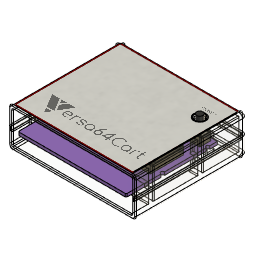
versa64case_2_0_closed v9 (Autodesk Fusion 360 design; units mm, degrees)
Autodesk Fusion 360 part; units mm, degrees
(part 1 of 2)
sketch "Versa64Cart_v1_6" plane through (0, 0, 0) normal (0, 0, 1) x (1, 0, 0) in component "Versa64cart_v1.6"
  line L0 (0, 11) -> (0, 18.6)
  line L1 (0, 20.6) -> (0, 42.9)
  line L2 (0, 44.9) -> (0, 48.9)
  line L3 (0, 48.9) -> (58, 48.9)
  line L4 (58, 48.9) -> (58, 44.8)
  line L5 (58, 42.9) -> (58, 20.6)
  line L6 (58, 18.6) -> (58, 11)
  arc A0 (0, 18.6) -> (1, 19.6) centre (0, 19.6) ccw
  arc A1 (1, 19.6) -> (0, 20.6) centre (0, 19.6) ccw
  arc A2 (0, 42.9) -> (1, 43.9) centre (0, 43.9) ccw
  arc A3 (1, 43.9) -> (0, 44.9) centre (0, 43.9) ccw
  arc A4 (57, 19.6) -> (58, 18.6) centre (58, 19.6) ccw
  arc A5 (58, 20.6) -> (57, 19.6) centre (58, 19.6) ccw
  line L7 (58, 42.9) -> (57.9, 42.9)
  arc A6 (57, 43.8) -> (57.9, 42.9) centre (57.9, 43.8) ccw
  arc A7 (58, 44.8) -> (57, 43.8) centre (58, 43.8) ccw
  circle A8 centre (29, 43.9) radius 2.5
  line L8 (57.5, 0) -> (0.5, 0)
  line L9 (0.5, 0) -> (0, 0.5)
  line L10 (0, 0.5) -> (0, 11)
  line L11 (57.5, 0) -> (58, 0.5)
  line L12 (58, 0.5) -> (58, 11)
  line L13 (19.4945, 23.3362) -> (19.4945, 18.0023) construction
  arc A9 (19.4945, 23.3363) -> (19.4945, 25.8763) centre (19.4945, 24.6063) ccw construction
  line L14 (54.8005, 18.0023) -> (54.8005, 31.2103) construction
  line L15 (19.4945, 31.2103) -> (19.4945, 25.8763) construction
  line L16 (19.4945, 31.2103) -> (54.8005, 31.2103) construction
  line L17 (19.4945, 18.0023) -> (54.8005, 18.0023) construction
  line L18 (41.7512, 46.99) -> (43.0213, 46.99)
  line L19 (43.0213, 46.99) -> (43.3388, 46.6725)
  line L20 (43.3388, 44.7675) -> (43.0213, 44.45)
  line L21 (41.1163, 46.355) -> (41.1163, 45.085)
  line L22 (41.7512, 46.99) -> (41.1163, 46.355)
  line L23 (41.1163, 45.085) -> (41.1163, 44.45)
  line L24 (43.0213, 44.45) -> (41.1163, 44.45)
  line L25 (43.9738, 46.6725) -> (44.2913, 46.99)
  line L26 (44.2913, 46.99) -> (45.5613, 46.99)
  line L27 (45.5613, 44.45) -> (44.2913, 44.45)
  line L28 (44.2913, 44.45) -> (43.9738, 44.7675)
  line L29 (44.2913, 46.99) -> (45.5613, 46.99)
  line L30 (45.5613, 46.99) -> (45.8788, 46.6725)
  line L31 (45.8788, 44.7675) -> (45.5613, 44.45)
  line L32 (46.5138, 46.6725) -> (46.8313, 46.99)
  line L33 (46.8313, 46.99) -> (48.1013, 46.99)
  line L34 (48.1013, 46.99) -> (48.7363, 46.355)
  line L35 (48.7363, 46.355) -> (48.7363, 45.085)
  line L36 (48.7363, 45.085) -> (48.1013, 44.45)
  line L37 (48.1013, 44.45) -> (46.8313, 44.45)
  line L38 (46.8313, 44.45) -> (46.5138, 44.7675)
  line L39 (40.64, 45.8788) -> (40.7988, 46.0375)
  line L40 (40.7988, 46.0375) -> (40.7988, 45.4025)
  line L41 (40.64, 45.4025) -> (40.9575, 45.4025)
  line L42 (40.64, 46.99) -> (40.64, 44.45)
  line L43 (40.005, 46.99) -> (38.735, 46.99)
  line L44 (40.64, 46.99) -> (40.005, 46.99)
  line L45 (38.735, 46.99) -> (38.1, 46.355)
  line L46 (38.1, 44.45) -> (38.1, 46.355)
  line L47 (40.64, 44.45) -> (40.64, 42.545)
  line L48 (40.64, 42.545) -> (40.005, 41.91)
  line L49 (40.005, 41.91) -> (38.735, 41.91)
  line L50 (38.735, 41.91) -> (38.1, 42.545)
  line L51 (38.1, 42.545) -> (38.1, 44.45)
  line L52 (38.1, 46.355) -> (38.1, 44.45)
  line L53 (37.465, 46.99) -> (36.195, 46.99)
  line L54 (38.1, 46.355) -> (37.465, 46.99)
  line L55 (36.195, 46.99) -> (35.56, 46.355)
  line L56 (35.56, 43.815) -> (35.56, 46.355)
  line L57 (38.1, 44.45) -> (38.1, 42.545)
  line L58 (38.1, 42.545) -> (37.465, 41.91)
  line L59 (37.465, 41.91) -> (36.195, 41.91)
  line L60 (36.195, 41.91) -> (35.56, 42.545)
  line L61 (35.56, 42.545) -> (35.56, 43.815)
  line L62 (34.925, 46.99) -> (33.655, 46.99)
  line L63 (35.56, 46.355) -> (34.925, 46.99)
  line L64 (33.655, 46.99) -> (33.02, 46.355)
  line L65 (33.02, 43.815) -> (33.02, 46.355)
  line L66 (35.56, 42.545) -> (34.925, 41.91)
  line L67 (34.925, 41.91) -> (33.655, 41.91)
  line L68 (33.655, 41.91) -> (33.02, 42.545)
  line L69 (33.02, 42.545) -> (33.02, 43.815)
  line L70 (1.6193, 35.8458) -> (15.8433, 35.8458)
  line L71 (15.8433, 45.7518) -> (1.6193, 45.7518)
  line L72 (1.6193, 45.7518) -> (1.6193, 42.4498)
  line L73 (1.6193, 39.1478) -> (2.1273, 39.1478)
  line L74 (2.1273, 39.1478) -> (2.1273, 42.4498)
  line L75 (2.1273, 42.4498) -> (1.6193, 42.4498)
  line L76 (1.6193, 39.1478) -> (1.6193, 35.8458)
  line L77 (1.6193, 42.4498) -> (1.6193, 39.1478)
  line L78 (15.8433, 35.8458) -> (15.8433, 39.1478)
  line L79 (15.8433, 42.4498) -> (15.3353, 42.4498)
  line L80 (15.3353, 42.4498) -> (15.3353, 39.1478)
  line L81 (15.3353, 39.1478) -> (15.8433, 39.1478)
  line L82 (15.8433, 42.4498) -> (15.8433, 45.7518)
  line L83 (15.8433, 39.1478) -> (15.8433, 42.4498)
  line L84 (2.8893, 41.6878) -> (2.8893, 38.8938)
  line L85 (4.4133, 38.8938) -> (4.4133, 41.6878)
  line L86 (4.4133, 38.8938) -> (2.8893, 38.8938)
  line L87 (3.1433, 40.7988) -> (3.1433, 39.1478)
  line L88 (4.1593, 40.7988) -> (4.1593, 39.1478)
  line L89 (2.8893, 42.4498) -> (2.8893, 42.7037)
  line L90 (2.8893, 42.7037) -> (3.1433, 42.7037)
  line L91 (4.1593, 42.7037) -> (4.4133, 42.7037)
  line L92 (4.4133, 42.7037) -> (4.4133, 42.4498)
  line L93 (5.4293, 41.6878) -> (5.4293, 38.8938)
  line L94 (6.9533, 38.8938) -> (6.9533, 41.6878)
  line L95 (6.9533, 38.8938) -> (5.4293, 38.8938)
  line L96 (5.6833, 40.7988) -> (5.6833, 39.1478)
  line L97 (6.6993, 40.7988) -> (6.6993, 39.1478)
  line L98 (5.4293, 42.4498) -> (5.4293, 42.7037)
  line L99 (5.4293, 42.7037) -> (5.6833, 42.7037)
  line L100 (6.6993, 42.7037) -> (6.9533, 42.7037)
  line L101 (6.9533, 42.7037) -> (6.9533, 42.4498)
  line L102 (7.9693, 41.6878) -> (7.9693, 38.8938)
  line L103 (9.4932, 38.8938) -> (9.4932, 41.6878)
  line L104 (9.4932, 38.8938) -> (7.9693, 38.8938)
  line L105 (8.2233, 40.7988) -> (8.2233, 39.1478)
  line L106 (9.2393, 40.7988) -> (9.2393, 39.1478)
  line L107 (7.9693, 42.4498) -> (7.9693, 42.7037)
  line L108 (7.9693, 42.7037) -> (8.2233, 42.7037)
  line L109 (9.2393, 42.7037) -> (9.4932, 42.7037)
  line L110 (9.4932, 42.7037) -> (9.4932, 42.4498)
  line L111 (10.5092, 41.6878) -> (10.5092, 38.8938)
  line L112 (12.0333, 38.8938) -> (12.0333, 41.6878)
  line L113 (12.0333, 38.8938) -> (10.5092, 38.8938)
  line L114 (10.7633, 40.7988) -> (10.7633, 39.1478)
  line L115 (11.7793, 40.7988) -> (11.7793, 39.1478)
  line L116 (10.5092, 42.4498) -> (10.5092, 42.7037)
  line L117 (10.5092, 42.7037) -> (10.7633, 42.7037)
  line L118 (11.7793, 42.7037) -> (12.0333, 42.7037)
  line L119 (12.0333, 42.7037) -> (12.0333, 42.4498)
  line L120 (13.0493, 41.6878) -> (13.0493, 38.8938)
  line L121 (14.5732, 38.8938) -> (14.5732, 41.6878)
  line L122 (14.5732, 38.8938) -> (13.0493, 38.8938)
  line L123 (13.3033, 40.7988) -> (13.3033, 39.1478)
  line L124 (14.3193, 40.7988) -> (14.3193, 39.1478)
  line L125 (13.0493, 42.4498) -> (13.0493, 42.7037)
  line L126 (13.0493, 42.7037) -> (13.3033, 42.7037)
  line L127 (14.3193, 42.7037) -> (14.5732, 42.7037)
  line L128 (14.5732, 42.7037) -> (14.5732, 42.4498)
  line L129 (55.65, 41.6) -> (50.15, 41.6)
  line L130 (49.9, 43.15) -> (49.9, 46)
  line L131 (50.5, 47.6) -> (55.65, 47.6)
  line L132 (55.9, 46.05) -> (55.9, 43.15)
  arc A10 (55.35, 47.15) -> (55.4, 46.4) centre (55.0498, 46.7533) ccw
  arc A11 (55.35, 42.85) -> (55.4, 42.1) centre (55.0498, 42.4533) ccw
  arc A12 (50.45, 42.05) -> (50.4, 42.8) centre (50.7502, 42.4467) ccw
  arc A13 (50.45, 46.35) -> (50.45, 47.15) centre (50.75, 46.75) ccw
  circle A14 centre (52.9, 44.6) radius 1.75
  circle A15 centre (52.9, 44.6) radius 1.4
  line L133 (9.2393, 39.7828) -> (9.2393, 40.1638)
  line L134 (5.6833, 39.7828) -> (6.6993, 39.7828)
  line L135 (4.1593, 40.1638) -> (3.1433, 40.1638)
  line L136 (5.6833, 40.4178) -> (6.6993, 40.4178)
  line L137 (11.7793, 39.1478) -> (11.7793, 39.5288)
  line L138 (6.6993, 40.1638) -> (5.6833, 40.1638)
  line L139 (3.1433, 39.5288) -> (3.1433, 39.1478)
  line L140 (4.1593, 40.7988) -> (3.1433, 40.7988)
  line L141 (8.2233, 39.7828) -> (9.2393, 39.7828)
  line L142 (11.7793, 39.7828) -> (11.7793, 40.1638)
  line L143 (10.7633, 40.4178) -> (11.7793, 40.4178)
  line L144 (3.1433, 40.7988) -> (3.1433, 40.4178)
  line L145 (6.6993, 40.4178) -> (6.6993, 40.7988)
  line L146 (6.6993, 39.5288) -> (5.6833, 39.5288)
  line L147 (9.2393, 40.1638) -> (8.2233, 40.1638)
  line L148 (6.6993, 40.7988) -> (5.6833, 40.7988)
  line L149 (11.7793, 40.1638) -> (10.7633, 40.1638)
  line L150 (11.7793, 40.7988) -> (10.7633, 40.7988)
  line L151 (9.2393, 40.4178) -> (9.2393, 40.7988)
  line L152 (9.2393, 39.5288) -> (8.2233, 39.5288)
  line L153 (3.1433, 39.1478) -> (4.1593, 39.1478)
  line L154 (4.1593, 40.4178) -> (4.1593, 40.7988)
  line L155 (10.7633, 39.7828) -> (11.7793, 39.7828)
  line L156 (3.1433, 40.4178) -> (4.1593, 40.4178)
  line L157 (11.7793, 40.4178) -> (11.7793, 40.7988)
  line L158 (3.1433, 40.1638) -> (3.1433, 39.7828)
  line L159 (13.3033, 40.1638) -> (13.3033, 39.7828)
  line L160 (10.7633, 39.5288) -> (10.7633, 39.1478)
  line L161 (8.2233, 40.7988) -> (8.2233, 40.4178)
  line L162 (13.3033, 39.7828) -> (14.3193, 39.7828)
  line L163 (14.3193, 40.1638) -> (13.3033, 40.1638)
  line L164 (8.2233, 39.5288) -> (8.2233, 39.1478)
  line L165 (14.3193, 39.5288) -> (13.3033, 39.5288)
  line L166 (5.6833, 40.7988) -> (5.6833, 40.4178)
  line L167 (4.1593, 39.1478) -> (4.1593, 39.5288)
  line L168 (8.2233, 39.1478) -> (9.2393, 39.1478)
  line L169 (13.3033, 39.5288) -> (13.3033, 39.1478)
  line L170 (3.1433, 39.7828) -> (4.1593, 39.7828)
  line L171 (11.7793, 39.5288) -> (10.7633, 39.5288)
  line L172 (13.3033, 39.1478) -> (14.3193, 39.1478)
  line L173 (14.3193, 39.7828) -> (14.3193, 40.1638)
  line L174 (9.2393, 39.1478) -> (9.2393, 39.5288)
  line L175 (13.3033, 40.4178) -> (14.3193, 40.4178)
  line L176 (14.3193, 40.4178) -> (14.3193, 40.7988)
  line L177 (14.3193, 39.1478) -> (14.3193, 39.5288)
  line L178 (14.3193, 40.7988) -> (13.3033, 40.7988)
  line L179 (13.3033, 40.7988) -> (13.3033, 40.4178)
  line L180 (9.2393, 40.7988) -> (8.2233, 40.7988)
  line L181 (8.2233, 40.1638) -> (8.2233, 39.7828)
  line L182 (10.7633, 39.1478) -> (11.7793, 39.1478)
  line L183 (5.6833, 40.1638) -> (5.6833, 39.7828)
  line L184 (10.7633, 40.1638) -> (10.7633, 39.7828)
  line L185 (6.6993, 39.7828) -> (6.6993, 40.1638)
  line L186 (8.2233, 40.4178) -> (9.2393, 40.4178)
  line L187 (5.6833, 39.5288) -> (5.6833, 39.1478)
  line L188 (5.6833, 39.1478) -> (6.6993, 39.1478)
  line L189 (10.7633, 40.7988) -> (10.7633, 40.4178)
  line L190 (6.6993, 39.1478) -> (6.6993, 39.5288)
  line L191 (4.1593, 39.5288) -> (3.1433, 39.5288)
  line L192 (4.1593, 39.7828) -> (4.1593, 40.1638)
  line L193 (55.9, 42.7) -> (55.9, 42)
  line L194 (34.036, 45.974) -> (34.036, 45.466)
  line L195 (45.1803, 45.974) -> (44.6723, 45.974)
  line L196 (36.576, 45.974) -> (36.576, 45.466)
  line L197 (36.576, 45.466) -> (37.084, 45.466)
  line L198 (42.1323, 45.466) -> (42.6403, 45.466)
  line L199 (47.2123, 45.466) -> (47.7203, 45.466)
  line L200 (49.9, 42) -> (49.9, 42.7)
  line L201 (49.4, 42.7) -> (49.4, 42)
  line L202 (49.4, 42) -> (49.9, 42)
  line L203 (56.4, 42) -> (56.4, 42.7)
  line L204 (56.4, 47.2) -> (55.9, 47.2)
  line L205 (56.4, 42.7) -> (55.9, 42.7)
  line L206 (36.576, 42.926) -> (37.084, 42.926)
  line L207 (39.116, 45.974) -> (39.116, 45.466)
  line L208 (55.9, 47.2) -> (55.9, 46.5)
  line L209 (55.9, 46.5) -> (56.4, 46.5)
  line L210 (56.4, 46.5) -> (56.4, 47.2)
  line L211 (49.9, 47.2) -> (49.4, 47.2)
  line L212 (49.4, 47.2) -> (49.4, 46.5)
  line L213 (34.544, 42.926) -> (34.544, 43.434)
  line L214 (47.2123, 45.974) -> (47.2123, 45.466)
  line L215 (39.116, 43.434) -> (39.116, 42.926)
  line L216 (37.084, 43.434) -> (36.576, 43.434)
  line L217 (42.1323, 45.974) -> (42.1323, 45.466)
  line L218 (36.576, 43.434) -> (36.576, 42.926)
  line L219 (34.544, 45.466) -> (34.544, 45.974)
  line L220 (39.116, 45.466) -> (39.624, 45.466)
  line L221 (39.624, 45.466) -> (39.624, 45.974)
  line L222 (39.624, 45.974) -> (39.116, 45.974)
  line L223 (34.544, 43.434) -> (34.036, 43.434)
  line L224 (37.084, 45.466) -> (37.084, 45.974)
  line L225 (34.036, 45.466) -> (34.544, 45.466)
  line L226 (34.036, 42.926) -> (34.544, 42.926)
  line L227 (34.036, 43.434) -> (34.036, 42.926)
  line L228 (39.624, 42.926) -> (39.624, 43.434)
  line L229 (49.9, 46.5) -> (49.9, 47.2)
  line L230 (49.4, 46.5) -> (49.9, 46.5)
  line L231 (55.9, 42) -> (56.4, 42)
  line L232 (49.9, 42.7) -> (49.4, 42.7)
  line L233 (39.624, 43.434) -> (39.116, 43.434)
  line L234 (37.084, 42.926) -> (37.084, 43.434)
  line L235 (37.084, 45.974) -> (36.576, 45.974)
  line L236 (47.7203, 45.974) -> (47.2123, 45.974)
  line L237 (44.6723, 45.974) -> (44.6723, 45.466)
  line L238 (39.116, 42.926) -> (39.624, 42.926)
  line L239 (47.7203, 45.466) -> (47.7203, 45.974)
  line L240 (45.1803, 45.466) -> (45.1803, 45.974)
  line L241 (42.6403, 45.466) -> (42.6403, 45.974)
  line L242 (34.544, 45.974) -> (34.036, 45.974)
  line L243 (42.6403, 45.974) -> (42.1323, 45.974)
  line L244 (44.6723, 45.466) -> (45.1803, 45.466)
  line L245 (43.3388, 46.6725) -> (43.6563, 46.355)
  line L246 (43.6563, 46.355) -> (43.6563, 45.085)
  line L247 (43.6563, 45.085) -> (43.3388, 44.7675)
  line L248 (43.6563, 46.355) -> (43.9738, 46.6725)
  line L249 (43.9738, 44.7675) -> (43.6563, 45.085)
  line L250 (45.8788, 46.6725) -> (46.1962, 46.355)
  line L251 (46.1962, 46.355) -> (46.1962, 45.085)
  line L252 (46.1962, 45.085) -> (45.8788, 44.7675)
  line L253 (46.1962, 46.355) -> (46.5138, 46.6725)
  line L254 (46.5138, 44.7675) -> (46.1962, 45.085)
  line L255 (2.8893, 42.4498) -> (2.8893, 41.6878)
  line L256 (4.4133, 42.4498) -> (4.4133, 41.6878)
  line L257 (3.1433, 42.7037) -> (4.1593, 42.7037)
  line L258 (5.4293, 42.4498) -> (5.4293, 41.6878)
  line L259 (6.9533, 42.4498) -> (6.9533, 41.6878)
  line L260 (5.6833, 42.7037) -> (6.6993, 42.7037)
  line L261 (7.9693, 42.4498) -> (7.9693, 41.6878)
  line L262 (9.4932, 42.4498) -> (9.4932, 41.6878)
  line L263 (8.2233, 42.7037) -> (9.2393, 42.7037)
  line L264 (10.5092, 42.4498) -> (10.5092, 41.6878)
  line L265 (12.0333, 42.4498) -> (12.0333, 41.6878)
  line L266 (10.7633, 42.7037) -> (11.7793, 42.7037)
  line L267 (13.0493, 42.4498) -> (13.0493, 41.6878)
  line L268 (14.5732, 42.4498) -> (14.5732, 41.6878)
  line L269 (13.3033, 42.7037) -> (14.3193, 42.7037)
  line L270 (3.4607, 37.7578) -> (3.8488, 38.0682)
  line L271 (3.8488, 38.0682) -> (3.8488, 36.6713)
  line L272 (3.4607, 36.6713) -> (4.2369, 36.6713)
  line L273 (2.4447, 43.7903) -> (2.4447, 44.4112)
  arc A16 (3.2209, 44.4112) -> (2.4447, 44.4112) centre (2.8328, 44.4112) ccw
  line L274 (3.2209, 44.4112) -> (3.2209, 43.7903)
  arc A17 (2.4447, 43.7903) -> (3.2209, 43.7903) centre (2.8328, 43.7903) ccw
  line L275 (3.8592, 43.4023) -> (3.8592, 44.7993)
  line L276 (3.8592, 44.7993) -> (4.6353, 43.4023)
  line L277 (4.6353, 43.4023) -> (4.6353, 44.7993)
  arc A18 (6.5229, 37.719) -> (6.1736, 38.0683) centre (6.1736, 37.719) ccw
  arc A19 (6.1736, 38.0683) -> (5.7467, 37.7578) centre (6.1736, 37.6196) ccw
  arc A20 (6.4064, 37.4474) -> (6.5228, 37.719) centre (6.1477, 37.719) ccw
  line L278 (6.4064, 37.4474) -> (5.7468, 36.6713)
  line L279 (5.7468, 36.6713) -> (6.5229, 36.6713)
  line L280 (8.2867, 36.6713) -> (8.6748, 36.6713)
  arc A21 (8.6748, 36.6712) -> (8.6748, 37.4474) centre (8.6748, 37.0593) ccw
  line L281 (8.2867, 38.0682) -> (8.7524, 38.0682)
  arc A22 (8.7524, 37.4474) -> (8.7524, 38.0682) centre (8.7524, 37.7578) ccw
  line L282 (8.7524, 37.4474) -> (8.442, 37.4474)
  line L283 (11.1372, 38.0682) -> (10.8268, 36.9817)
  line L284 (10.8268, 36.9817) -> (11.6029, 36.9817)
  line L285 (11.37, 37.2921) -> (11.37, 36.6713)
  line L286 (13.3668, 36.6713) -> (13.8324, 36.6713)
  arc A23 (13.8324, 36.6713) -> (14.1428, 36.9817) centre (13.8324, 36.9817) ccw
  line L287 (14.1429, 36.9817) -> (14.1429, 37.1369)
  arc A24 (14.1428, 37.1369) -> (13.8324, 37.4473) centre (13.8324, 37.1369) ccw
  line L288 (13.8324, 37.4474) -> (13.3668, 37.4474)
  line L289 (13.3668, 37.4474) -> (13.3668, 38.0682)
  line L290 (13.3668, 38.0682) -> (14.1429, 38.0682)
  line L291 (55.9, 43.15) -> (55.9, 41.8)
  arc A25 (55.7, 41.6) -> (55.9, 41.8) centre (55.7, 41.8) ccw
  line L292 (55.7, 41.6) -> (55.65, 41.6)
  line L293 (50.15, 41.6) -> (50.1, 41.6)
  arc A26 (49.9, 41.8) -> (50.1, 41.6) centre (50.1, 41.8) ccw
  line L294 (49.9, 41.8) -> (49.9, 43.15)
  line L295 (49.9, 46) -> (49.9, 47.4)
  arc A27 (50.1, 47.6) -> (49.9, 47.4) centre (50.1, 47.4) ccw
  line L296 (50.1, 47.6) -> (50.5, 47.6)
  line L297 (55.65, 47.6) -> (55.7, 47.6)
  arc A28 (55.9, 47.4) -> (55.7, 47.6) centre (55.7, 47.4) ccw
  line L298 (55.9, 47.4) -> (55.9, 46.05)
  arc A29 (55.4, 46.4) -> (55.35, 47.15) centre (55.0498, 46.7533) ccw
  arc A30 (55.4, 42.1) -> (55.35, 42.85) centre (55.0498, 42.4533) ccw
  arc A31 (50.4, 42.8) -> (50.45, 42.05) centre (50.7502, 42.4467) ccw
  arc A32 (50.45, 47.15) -> (50.45, 46.35) centre (50.75, 46.75) ccw
  line L299 (19.4945, 31.2103) -> (54.8005, 18.0023) construction
  line L300 (55.1475, 33.5063) -> (19.1475, 33.5063)
  line L301 (19.1475, 15.7063) -> (55.1475, 15.7063)
  line L302 (55.1475, 15.7063) -> (55.1475, 33.5063)
  line L303 (55.1475, 33.5063) -> (19.1475, 15.7063) construction
  line L304 (19.1475, 33.5063) -> (55.1475, 15.7063) construction
  arc A33 (19.1475, 23.3563) -> (19.1475, 25.8563) centre (19.1475, 24.6063) ccw
  line L305 (19.1475, 33.5063) -> (19.1475, 25.8563)
  line L306 (19.1475, 23.3563) -> (19.1475, 15.7063)
  line L307 (55.5475, 31.2063) -> (18.7475, 31.2063)
  line L308 (18.7475, 18.0063) -> (55.5475, 18.0063)
  line L309 (55.5475, 18.0063) -> (55.5475, 31.2063)
  line L310 (55.5475, 31.2063) -> (18.7475, 18.0063) construction
  line L311 (18.7475, 31.2063) -> (55.5475, 18.0063) construction
  arc A34 (18.7475, 23.8563) -> (18.7475, 25.3563) centre (18.7475, 24.6063) ccw
  line L312 (18.7475, 31.2063) -> (18.7475, 25.3563)
  line L313 (18.7475, 23.8563) -> (18.7475, 18.0063)
  point P0 (37.1475, 24.6063)
  point P1 (37.1475, 24.6063)
  dimension "d25" = 36
  dimension "d26" = 17.8
  dimension "d28" = 1.25
  dimension "d29" = 36.8
  dimension "d30" = 13.2
  dimension "d32" = 0.75
  constraint horizontal L300
  constraint perpendicular L300 L305
  constraint parallel L300 L301
  constraint parallel L302 L305
  constraint coincident L303 P1
  constraint coincident L304 P1
  constraint midpoint L299 P1
  constraint coincident A33.start L305
  constraint collinear L305 L306
  constraint coincident A33.centre L305
  constraint horizontal L307
  constraint perpendicular L307 L312
  constraint parallel L307 L308
  constraint parallel L309 L312
  constraint coincident L310 P1
  constraint coincident L311 P1
  constraint coincident P1 P0
  constraint coincident A34.start L312
  constraint collinear L312 L313
  constraint coincident A34.centre L312
  measures "d25" distance of L301.start L301.end
  measures "d26" distance of L300.end L301.start
  measures "d28" radius of A33
  measures "d29" distance of L308.start L308.end
  measures "d30" distance of L307.end L308.start
  measures "d32" radius of A34
  measures "d122" radius of L2.start
  measures "d233" radius of L2.start
extrude "Extrude1" add sketch "Versa64Cart_v1_6" against normal blind 1.6 contours L0 L1 L2 L3 L4 L5 L6 A0 A1 A2 A3 A4 A5 L7 A6 A7 L8 L9 L10 L11 L12 | L18 L19 L20 L21 L22 L23 L24 L245 L246 L247 | L25 L26 L27 L28 L29 L30 L31 L246 L248 L249 L250 L251 L252 | L32 L33 L34 L35 L36 L37 L38 L251 L253 L254 | L42 L43 L44 L45 L46 L47 L48 L49 L50 L51 L52 L57 | L39 L40 L41 L42 | L46 L51 L52 L53 L54 L55 L56 L57 L58 L59 L60 L61 | L56 L61 L62 L63 L64 L65 L66 L67 L68 L69 | L70 L71 L72 L73 L74 L75 L76 L78 L79 L80 L81 L82 | L73 L74 L75 L77 | L79 L80 L81 L83 | L84 L85 L86 L89 L90 L91 L92 L255 L256 L257 | L87 L88 L140 L144 L154 L156 | L87 L88 L135 L156 | L87 L88 L135 L158 L170 L192 | L87 L88 L170 L191 | L87 L88 L139 L153 L167 L191 | L93 L94 L95 L98 L99 L100 L101 L258 L259 L260 | L96 L97 L136 L145 L148 L166 | L96 L97 L136 L138 | L96 L97 L134 L138 L183 L185 | L96 L97 L134 L146 | L96 L97 L146 L187 L188 L190 | L102 L103 L104 L107 L108 L109 L110 L261 L262 L263 | L105 L106 L151 L161 L180 L186 | L105 L106 L147 L186 | L105 L106 L133 L141 L147 L181 | L105 L106 L141 L152 | L105 L106 L152 L164 L168 L174 | L111 L112 L113 L116 L117 L118 L119 L264 L265 L266 | L114 L115 L143 L150 L157 L189 | L114 L115 L143 L149 | L114 L115 L142 L149 L155 L184 | L114 L115 L155 L171 | L114 L115 L137 L160 L171 L182 | L120 L121 L122 L125 L126 L127 L128 L267 L268 L269 | L123 L124 L175 L176 L178 L179 | L123 L124 L163 L175 | L123 L124 L159 L162 L163 L173 | L123 L124 L162 L165 | L123 L124 L165 L169 L172 L177 | L129 L130 L131 L132 L193 L200 L208 L229 L291 A25 L292 L293 A26 L294 L295 A27 L296 L297 A28 L298 | L193 L203 L205 L231 L291 | L200 L201 L202 L232 L294 | L204 L208 L209 L210 L298 | L211 L212 L229 L230 L295 | A10 A29 | A11 A30 | A12 A31 | A13 A32 | A14 | A15 | L194 L219 L225 L242 | L195 L237 L240 L244 | L196 L197 L224 L235 | L198 L217 L241 L243 | L199 L214 L236 L239 | L206 L216 L218 L234 | L207 L220 L221 L222 | L213 L223 L226 L227 | L215 L228 L233 L238 | L273 A16 L274 A17 | L300 L302 L305 L307 | L302 L307 L308 L309 | L302 A33 L305 L306 L307 L308 | A33 L305 L306 L307 L308 A34 L312 L313 | L301 L302 L306 L308 makes body 1 in component "Versa64cart_v1.6"
extrude "Extrude2" add sketch "Versa64Cart_v1_6" along normal blind 5.3 contours L70 L71 L72 L73 L74 L75 L76 L78 L79 L80 L81 L82 | L273 A16 L274 A17 bodies 1 in component "Versa64cart_v1.6"
extrude "Extrude4" add sketch "Versa64Cart_v1_6" along normal blind 7 contours L87 L88 L140 L144 L154 L156 | L87 L88 L135 L156 | L87 L88 L135 L158 L170 L192 | L87 L88 L170 L191 | L87 L88 L139 L153 L167 L191 | L96 L97 L136 L145 L148 L166 | L96 L97 L136 L138 | L96 L97 L134 L138 L183 L185 | L96 L97 L134 L146 | L96 L97 L146 L187 L188 L190 | L105 L106 L151 L161 L180 L186 | L105 L106 L147 L186 | L105 L106 L133 L141 L147 L181 | L105 L106 L141 L152 | L105 L106 L152 L164 L168 L174 | L114 L115 L143 L150 L157 L189 | L114 L115 L143 L149 | L114 L115 L142 L149 L155 L184 | L114 L115 L155 L171 | L114 L115 L137 L160 L171 L182 | L123 L124 L175 L176 L178 L179 | L123 L124 L163 L175 | L123 L124 L159 L162 L163 L173 | L123 L124 L162 L165 | L123 L124 L165 L169 L172 L177 bodies 1 in component "Versa64cart_v1.6"
extrude "Extrude5" add sketch "Versa64Cart_v1_6" along normal blind 4.5 contours L84 L85 L86 L89 L90 L91 L92 L255 L256 L257 | L93 L94 L95 L98 L99 L100 L101 L258 L259 L260 | L102 L103 L104 L107 L108 L109 L110 L261 L262 L263 | L111 L112 L113 L116 L117 L118 L119 L264 L265 L266 | L120 L121 L122 L125 L126 L127 L128 L267 L268 L269 bodies 1 in component "Versa64cart_v1.6"
extrude "Extrude6" add sketch "Versa64Cart_v1_6" along normal blind 9.5 contours L194 L219 L225 L242 | L195 L237 L240 L244 | L196 L197 L224 L235 | L198 L217 L241 L243 | L199 L214 L236 L239 | L206 L216 L218 L234 | L207 L220 L221 L222 | L213 L223 L226 L227 | L215 L228 L233 L238 bodies 1 in component "Versa64cart_v1.6"
extrude "Extrude7" add sketch "Versa64Cart_v1_6" along normal blind 2.5 contours L18 L19 L20 L21 L22 L23 L24 L245 L246 L247 | L25 L26 L27 L28 L29 L30 L31 L246 L248 L249 L250 L251 L252 | L32 L33 L34 L35 L36 L37 L38 L251 L253 L254 | L42 L43 L44 L45 L46 L47 L48 L49 L50 L51 L52 L57 | L46 L51 L52 L53 L54 L55 L56 L57 L58 L59 L60 L61 | L56 L61 L62 L63 L64 L65 L66 L67 L68 L69 bodies 1 in component "Versa64cart_v1.6"
extrude "Extrude8" add sketch "Versa64Cart_v1_6" along normal blind 4.5 contours L129 L130 L131 L132 L193 L200 L208 L229 L291 A25 L292 L293 A26 L294 L295 A27 L296 L297 A28 L298 bodies 1 in component "Versa64cart_v1.6"
extrude "Extrude9" add sketch "Versa64Cart_v1_6" along normal blind 4.7 contours A10 A29 | A11 A30 | A12 A31 | A13 A32 bodies 1 in component "Versa64cart_v1.6"
extrude "Extrude10" add sketch "Versa64Cart_v1_6" along normal blind 12.5 contours A14 | A15 bodies 1 in component "Versa64cart_v1.6"
extrude "Extrude11" add sketch "Versa64Cart_v1_6" along normal blind 4.3 contours L300 L302 L305 L307 | L302 A33 L305 L306 L307 L308 | L301 L302 L306 L308 bodies 1 in component "Versa64cart_v1.6"
extrude "Extrude12" add sketch "Versa64Cart_v1_6" along normal blind 4.7 from surface at 4.3 contours L302 L307 L308 L309 | L302 A33 L305 L306 L307 L308 | A33 L305 L306 L307 L308 A34 L312 L313 bodies 1 in component "Versa64cart_v1.6"
chamfer "Chamfer1" distance 0.15 angle 45 36 edges at (34.29, 42.926, 9.5) (34.544, 43.18, 9.5) (34.29, 43.434, 9.5) (34.036, 43.18, 9.5) (34.036, 45.72, 9.5) (34.29, 45.974, 9.5) (34.544, 45.72, 9.5) (34.29, 45.466, 9.5) (36.576, 43.18, 9.5) (36.83, 43.434, 9.5) (36.83, 42.926, 9.5) (37.084, 43.18, 9.5) (36.576, 45.72, 9.5) (36.83, 45.974, 9.5) (36.83, 45.466, 9.5) (37.084, 45.72, 9.5) (39.37, 43.434, 9.5) (39.37, 42.926, 9.5) (39.116, 43.18, 9.5) (39.624, 43.18, 9.5) (39.37, 45.466, 9.5) (39.116, 45.72, 9.5) (39.37, 45.974, 9.5) (39.624, 45.72, 9.5) (42.6403, 45.72, 9.5) (42.3863, 45.466, 9.5) (42.1323, 45.72, 9.5) (42.3863, 45.974, 9.5) (44.9263, 45.974, 9.5) (45.1803, 45.72, 9.5) (44.9263, 45.466, 9.5) (44.6723, 45.72, 9.5) (47.4663, 45.974, 9.5) (47.7203, 45.72, 9.5) (47.4663, 45.466, 9.5) (47.2123, 45.72, 9.5) on bodies 1 in component "Versa64cart_v1.6"
ref_plane "WorkPlane1" through (29, 24.45, 8.8) normal (0, 0, 1) x (1, 0, 0) in component "Versa64case_v2_top_closed"
sketch "Sketch1" plane through (0, 0, 8.8) normal (0, 0, 1) x (1, 0, 0) in component "Versa64case_v2_top_closed"
  line L0 (0, 48.9) -> (58, 48.9) construction
  line L1 (0, 44.9) -> (0, 48.9) construction
  arc A0 (0, 42.9) -> (0, 44.9) centre (0, 43.9) ccw construction
  line L2 (0, 20.6) -> (0, 42.9) construction
  arc A1 (0, 18.6) -> (0, 20.6) centre (0, 19.6) ccw construction
  line L3 (0, 0.5) -> (0, 18.6) construction
  line L4 (57.5, 0) -> (0.5, 0) construction
  line L5 (0.5, 0) -> (0, 0.5) construction
  line L6 (57.5, 0) -> (58, 0.5) construction
  line L7 (58, 0.5) -> (58, 18.6) construction
  arc A2 (58, 20.6) -> (58, 18.6) centre (58, 19.6) ccw construction
  line L8 (58, 42.9) -> (58, 20.6) construction
  arc A3 (57, 43.8) -> (57.9, 42.9) centre (57.9, 43.8) ccw construction
  arc A4 (58, 44.8) -> (57, 43.8) centre (58, 43.8) ccw construction
  line L9 (58, 48.9) -> (58, 44.8) construction
  circle A5 centre (52.9, 44.6) radius 1.75 construction
  line L10 (40.64, 46.99) -> (38.735, 46.99) construction
  line L11 (40.64, 42.545) -> (40.64, 46.99) construction
  line L12 (33.655, 41.91) -> (34.925, 41.91) construction
  line L13 (33.02, 46.355) -> (33.02, 42.545) construction
  line L14 (41.1163, 46.355) -> (41.1163, 44.45) construction
  line L15 (41.1163, 44.45) -> (43.0213, 44.45) construction
  line L16 (48.1013, 46.99) -> (46.8313, 46.99) construction
  line L17 (48.7363, 45.085) -> (48.7363, 46.355) construction
  circle A6 centre (29, 43.9) radius 2.5 construction
  line L18 (15.8433, 45.7518) -> (1.6193, 45.7518) construction
  line L19 (1.6193, 45.7518) -> (1.6193, 42.4498) construction
  line L20 (1.6193, 39.1478) -> (1.6193, 35.8458) construction
  line L21 (1.6193, 35.8458) -> (15.8433, 35.8458) construction
  line L22 (15.8433, 35.8458) -> (15.8433, 39.1478) construction
  line L23 (15.8433, 42.4498) -> (15.8433, 45.7518) construction
  line L24 (55.5475, 31.2063) -> (18.7475, 31.2063) construction
  line L25 (18.7475, 31.2063) -> (18.7475, 25.3563) construction
  arc A7 (18.7475, 23.8563) -> (18.7475, 25.3563) centre (18.7475, 24.6063) ccw construction
  line L26 (18.7475, 23.8563) -> (18.7475, 18.0063) construction
  line L27 (18.7475, 18.0063) -> (55.5475, 18.0063) construction
  line L28 (55.5475, 18.0063) -> (55.5475, 31.2063) construction
  line L29 (-2.5, 57.9) -> (60.5, 57.9)
  line L30 (61, 57.4) -> (61, 0)
  line L31 (61, 0) -> (-3, 0)
  line L32 (-3, 0) -> (-3, 57.4)
  circle A8 centre (29, 43.9) radius 3
  circle A9 centre (29, 43.9) radius 1.25
  circle A10 centre (52.9, 44.6) radius 2.25
  line L33 (18.7475, 31.7063) -> (55.5475, 31.7063)
  line L34 (56.0475, 31.2063) -> (56.0475, 18.0063)
  line L35 (55.5475, 17.5063) -> (18.7475, 17.5063)
  line L36 (18.2475, 18.0063) -> (18.2475, 31.2063)
  arc A11 (18.7475, 31.7063) -> (18.2475, 31.2063) centre (18.7475, 31.2063) ccw
  arc A12 (56.0475, 31.2063) -> (55.5475, 31.7063) centre (55.5475, 31.2063) ccw
  arc A13 (55.5475, 17.5063) -> (56.0475, 18.0063) centre (55.5475, 18.0063) ccw
  arc A14 (18.2475, 18.0063) -> (18.7475, 17.5063) centre (18.7475, 18.0063) ccw
  line L37 (-3, 9.5) -> (61, 9.5)
  line L38 (-3, 11.5) -> (61, 11.5)
  arc A15 (-2.5, 57.9) -> (-3, 57.4) centre (-2.5, 57.4) ccw
  arc A16 (61, 57.4) -> (60.5, 57.9) centre (60.5, 57.4) ccw
  line L39 (-2.5, 59.9) -> (60.5, 59.9)
  line L40 (63, 57.4) -> (63, 0)
  line L41 (63, 0) -> (-5, 0)
  line L42 (-5, 0) -> (-5, 57.4)
  arc A17 (63, 57.4) -> (60.5, 59.9) centre (60.5, 57.4) ccw
  arc A18 (-2.5, 59.9) -> (-5, 57.4) centre (-2.5, 57.4) ccw
  line L43 (-3, 35.3) -> (1.5, 35.3)
  line L44 (2, 34.8) -> (2, 33.8)
  line L45 (1.5, 33.3) -> (-3, 33.3)
  line L46 (-3, 33.3) -> (-3, 35.3)
  arc A19 (2, 34.8) -> (1.5, 35.3) centre (1.5, 34.8) ccw
  arc A20 (1.5, 33.3) -> (2, 33.8) centre (1.5, 33.8) ccw
  line L47 (56.5, 37.9) -> (61, 37.9)
  line L48 (61, 37.9) -> (61, 35.9)
  line L49 (61, 35.9) -> (56.5, 35.9)
  line L50 (56, 36.4) -> (56, 37.4)
  arc A21 (56.5, 37.9) -> (56, 37.4) centre (56.5, 37.4) ccw
  arc A22 (56, 36.4) -> (56.5, 35.9) centre (56.5, 36.4) ccw
  arc A23 (-2.5, 58.76) -> (-3.86, 57.4) centre (-2.5, 57.4) ccw
  line L51 (-3.86, 0) -> (-3.86, 57.4)
  line L52 (61.86, 57.4) -> (61.86, 0)
  arc A24 (61.86, 57.4) -> (60.5, 58.76) centre (60.5, 57.4) ccw
  line L53 (-2.5, 58.76) -> (60.5, 58.76)
  circle A25 centre (29, 43.9) radius 2.2
  line L54 (-0.3, 11.5) -> (-0.3, 9.5)
  line L55 (58.3, 11.5) -> (58.3, 9.5)
  line L56 (58.3, 37.9) -> (58.3, 35.9)
  line L57 (-0.3, 35.3) -> (-0.3, 33.3)
  line L58 (32, 43.9) -> (32, 57.9)
  line L59 (26, 43.9) -> (26, 54.9)
  arc A26 (26, 54.9) -> (23, 57.9) centre (23, 54.9) ccw
  line L60 (33.02, 47.29) -> (48.7363, 47.29)
  line L61 (49.0363, 46.99) -> (49.0363, 44.45)
  line L62 (48.7363, 44.15) -> (41.24, 44.15)
  line L63 (40.94, 43.85) -> (40.94, 41.91)
  line L64 (40.64, 41.61) -> (33.02, 41.61)
  line L65 (32.72, 41.91) -> (32.72, 46.99)
  arc A27 (49.0363, 46.99) -> (48.7363, 47.29) centre (48.7363, 46.99) ccw
  arc A28 (48.7363, 44.15) -> (49.0363, 44.45) centre (48.7363, 44.45) ccw
  arc A29 (41.24, 44.15) -> (40.94, 43.85) centre (41.24, 43.85) ccw
  arc A30 (40.64, 41.61) -> (40.94, 41.91) centre (40.64, 41.91) ccw
  arc A31 (32.72, 41.91) -> (33.02, 41.61) centre (33.02, 41.91) ccw
  arc A32 (33.02, 47.29) -> (32.72, 46.99) centre (33.02, 46.99) ccw
  dimension "d45" = 3
  dimension "d46" = 3
  dimension "d48" = 9
  dimension "d72" = 2.5
  dimension "d73" = 4.5
  dimension "d75" = 6
  dimension "d76" = 0.5
  dimension "d77" = 0.5
  dimension "d78" = 0.5
  dimension "d79" = 0.5
  dimension "d80" = 0.5
  dimension "d81" = 0.5
  dimension "d82" = 0.5
  dimension "d83" = 0.5
  dimension "d87" = 9.5
  dimension "d90" = 0.5
  dimension "d91" = 0.5
  dimension "d93" = 2
  dimension "d94" = 2
  dimension "d95" = 2
  dimension "d96" = 2.5
  dimension "d97" = 2.5
  dimension "d98" = 2
  dimension "d99" = 2
  dimension "d100" = 0.5
  dimension "d101" = 0.5
  dimension "d104" = 2
  dimension "d105" = 2
  dimension "d106" = 0.5
  dimension "d107" = 0.5
  dimension "d108" = 11
  dimension "d125" = 0.3
  dimension "d141" = 0.3
  dimension "d142" = 0.3
  dimension "d158" = 0.3
  dimension "d159" = 0.3
  dimension "d183" = 0.86
  dimension "d184" = 0.86
  dimension "d185" = 2
  dimension "d225" = 13.6
  dimension "d227" = 3
  dimension "d238" = 0.3
  dimension "d239" = 0.3
  dimension "d240" = 0.3
  dimension "d241" = 0.3
  dimension "d242" = 0.3
  dimension "d243" = 0.3
  dimension "d244" = 0.3
  dimension "d245" = 0.3
  dimension "d246" = 0.3
  dimension "d247" = 0.3
  dimension "d248" = 0.3
  dimension "d249" = 0.3
  constraint horizontal L29
  constraint vertical L30
  constraint horizontal L31
  constraint vertical L32
  constraint collinear L4 L31
  constraint concentric A6 A8
  constraint concentric A6 A9
  constraint concentric A5 A10
  constraint horizontal L33
  constraint vertical L34
  constraint horizontal L35
  constraint vertical L36
  constraint tangent L33 A11
  constraint tangent L36 A11
  constraint tangent L33 A12
  constraint tangent L34 A12
  constraint tangent L34 A13
  constraint tangent L35 A13
  constraint tangent L36 A14
  constraint tangent L35 A14
  constraint coincident L32 L37.start
  constraint coincident L30 L37.end
  constraint perpendicular L30 L37
  constraint coincident L32 L38.start
  constraint coincident L30 L38.end
  constraint perpendicular L30 L38
  constraint tangent L29 A15
  constraint tangent L32 A15
  constraint tangent L29 A16
  constraint tangent L30 A16
  constraint horizontal L39
  constraint vertical L40
  constraint horizontal L41
  constraint vertical L42
  constraint collinear L31 L41
  constraint tangent L39 A17
  constraint tangent L40 A17
  constraint tangent L39 A18
  constraint tangent L42 A18
  constraint horizontal L43
  constraint vertical L44
  constraint horizontal L45
  constraint vertical L46
  constraint coincident L32 L43.start
  constraint tangent L43 A19
  constraint tangent L44 A19
  constraint tangent L44 A20
  constraint tangent L45 A20
  constraint horizontal L47
  constraint vertical L48
  constraint horizontal L49
  constraint vertical L50
  constraint coincident L30 L48.end
  constraint tangent L50 A21
  constraint tangent L47 A21
  constraint tangent L50 A22
  constraint tangent L49 A22
  constraint concentric A15 A23
  constraint concentric A16 A24
  constraint tangent A23 L53
  constraint tangent A24 L53
  constraint tangent L52 A24
  constraint tangent A23 L51
  constraint coincident L41 L51.start
  constraint coincident L41 L52.end
  constraint concentric A9 A25
  constraint coincident L38 L54.start
  constraint coincident L37 L54.end
  constraint perpendicular L37 L54
  constraint coincident L38 L55.start
  constraint coincident L37 L55.end
  constraint perpendicular L37 L55
  constraint coincident L47 L56.start
  constraint coincident L49 L56.end
  constraint perpendicular L49 L56
  constraint coincident L43 L57.start
  constraint coincident L45 L57.end
  constraint perpendicular L45 L57
  constraint coincident L29 L58.end
  constraint perpendicular L29 L58
  constraint perpendicular L29 L59
  constraint tangent A8 L58
  constraint tangent A8 L59
  constraint coincident A8 L58.start
  constraint coincident A8 L59.start
  constraint tangent L59 A26
  constraint tangent L29 A26
  constraint coincident L29 A26.end
  constraint parallel L16 L60
  constraint perpendicular L16 L61
  constraint perpendicular L61 L62
  constraint perpendicular L62 L63
  constraint perpendicular L61 L64
  constraint perpendicular L60 L65
  constraint tangent L60 A27
  constraint tangent L61 A27
  constraint tangent L61 A28
  constraint tangent L62 A28
  constraint tangent L62 A29
  constraint tangent L63 A29
  constraint tangent L63 A30
  constraint tangent L64 A30
  constraint tangent L64 A31
  constraint tangent L65 A31
  constraint tangent L65 A32
  constraint tangent L60 A32
  measures "d45" distance of L1 L32
  measures "d46" distance of L9 L30
  measures "d48" distance of L0 L29
  measures "d72" diameter of A9
  measures "d73" diameter of A10
  measures "d75" diameter of A8
  measures "d76" distance of L25 L36
  measures "d77" distance of L28 L34
  measures "d78" distance of L24 L33
  measures "d79" distance of L27 L35
  measures "d80" radius of A11
  measures "d81" radius of A12
  measures "d82" radius of A13
  measures "d83" radius of A14
  measures "d87" distance of L31 L37
  measures "d90" radius of A15
  measures "d91" radius of A16
  measures "d93" distance of L32 L42
  measures "d94" distance of L30 L40
  measures "d95" distance of L29 L39
  measures "d96" radius of A17
  measures "d97" radius of A18
  measures "d98" distance of L43 L45
  measures "d99" distance of L2 L44
  measures "d100" radius of A19
  measures "d101" radius of A20
  measures "d104" distance of L47 L49
  measures "d105" distance of L8 L50
  measures "d106" radius of A21
  measures "d107" radius of A22
  measures "d108" distance of L0 L47
  measures "d125" distance of A6 A25
  measures "d141" distance of L3 L54
  measures "d142" distance of L7 L55
  measures "d158" distance of L2 L57
  measures "d159" distance of L8 L56
  measures "d183" distance of L32 L51
  measures "d184" distance of L30 L52
  measures "d185" distance of L37 L38
  measures "d225" distance of L0 L43
  measures "d227" radius of A26
  measures "d238" distance of L10 L60
  measures "d239" distance of L13 L65
  measures "d240" distance of L12 L64
  measures "d241" distance of L11 L63
  measures "d242" distance of L15 L62
  measures "d243" distance of L17 L61
  measures "d244" radius of A27
  measures "d245" radius of A28
  measures "d246" radius of A29
  measures "d247" radius of A30
  measures "d248" radius of A31
  measures "d249" radius of A32
ref_plane "WorkPlane1" through (29, 24.45, -8.1) normal (0, 0, -1) x (-1, 0, 0) in component "versa64case_v2_bottom_closed"
sketch "Sketch1 (2)" plane through (0, 0, -8.1) normal (0, 0, -1) x (-1, 0, 0) in component "versa64case_v2_bottom_closed"
  line L0 (0, 0.5) -> (0, 18.6) construction
  line L1 (0, 20.6) -> (0, 42.9) construction
  line L2 (-58, 0.5) -> (-58, 18.6) construction
  line L3 (-58, 42.9) -> (-58, 20.6) construction
  line L4 (0, 48.9) -> (-58, 48.9) construction
  circle A0 centre (-29, 43.9) radius 1.25 construction
  line L5 (3, 9.5) -> (-61, 9.5)
  line L6 (3, 11.5) -> (-61, 11.5)
  line L7 (3, 0) -> (3, 57.4)
  line L8 (5, 0) -> (5, 57.4)
  line L9 (-63, 0) -> (5, 0)
  line L10 (-63, 57.4) -> (-63, 0)
  line L11 (-61, 57.4) -> (-61, 0)
  arc A1 (5, 57.4) -> (2.5, 59.9) centre (2.5, 57.4) ccw
  arc A2 (3, 57.4) -> (2.5, 57.9) centre (2.5, 57.4) ccw
  line L12 (2.5, 57.9) -> (-60.5, 57.9)
  line L13 (2.5, 59.9) -> (-60.5, 59.9)
  arc A3 (-60.5, 59.9) -> (-63, 57.4) centre (-60.5, 57.4) ccw
  arc A4 (-60.5, 57.9) -> (-61, 57.4) centre (-60.5, 57.4) ccw
  line L14 (3, 35.3) -> (-1.5, 35.3)
  arc A5 (-1.5, 35.3) -> (-2, 34.8) centre (-1.5, 34.8) ccw
  line L15 (-2, 34.8) -> (-2, 33.8)
  arc A6 (-2, 33.8) -> (-1.5, 33.3) centre (-1.5, 33.8) ccw
  line L16 (-1.5, 33.3) -> (3, 33.3)
  line L17 (-56.5, 37.9) -> (-61, 37.9)
  arc A7 (-56, 37.4) -> (-56.5, 37.9) centre (-56.5, 37.4) ccw
  line L18 (-56, 36.4) -> (-56, 37.4)
  arc A8 (-56.5, 35.9) -> (-56, 36.4) centre (-56.5, 36.4) ccw
  line L19 (-61, 35.9) -> (-56.5, 35.9)
  line L20 (-58.3, 37.9) -> (-58.3, 35.9)
  line L21 (0.3, 35.3) -> (0.3, 33.3)
  circle A9 centre (-29, 43.9) radius 4
  circle A10 centre (-29, 43.9) radius 2.5 construction
  circle A11 centre (-29, 43.9) radius 1.6
  line L22 (-29, 43.9) -> (-29, 48.9) construction
  line L23 (-29, 43.9) -> (-33, 43.9) construction
  line L24 (-33, 43.9) -> (-33, 50.7)
  line L25 (-25, 43.9) -> (-25, 50.7)
  line L26 (-25.5, 51.2) -> (-32.5, 51.2)
  line L27 (-25, 49.2) -> (-33, 49.2)
  arc A12 (-25, 50.7) -> (-25.5, 51.2) centre (-25.5, 50.7) ccw
  arc A13 (-32.5, 51.2) -> (-33, 50.7) centre (-32.5, 50.7) ccw
  line L28 (-62.14, 0) -> (-62.14, 57.34)
  line L29 (2.44, 59.04) -> (-60.44, 59.04)
  line L30 (4.14, 0) -> (4.14, 57.34)
  arc A14 (4.14, 57.34) -> (2.44, 59.04) centre (2.44, 57.34) ccw
  arc A15 (-60.44, 59.04) -> (-62.14, 57.34) centre (-60.44, 57.34) ccw
  circle A16 centre (-29, 43.9) radius 2.35
  line L31 (-5, 49.2) -> (-13, 49.2)
  line L32 (-13, 49.2) -> (-13, 51.7)
  line L33 (-12.5, 52.2) -> (-5.5, 52.2)
  line L34 (-5, 51.7) -> (-5, 49.2)
  line L35 (-5, 49.2) -> (-13, 49.2)
  line L36 (-13, 49.2) -> (-13, 48.4)
  line L37 (-12.5, 47.9) -> (-5.5, 47.9)
  line L38 (-5, 48.4) -> (-5, 49.2)
  line L39 (0, 48.9) -> (-58, 48.9)
  line L40 (0, 44.9) -> (0, 48.9)
  arc A17 (-5, 51.7) -> (-5.5, 52.2) centre (-5.5, 51.7) ccw
  arc A18 (-12.5, 52.2) -> (-13, 51.7) centre (-12.5, 51.7) ccw
  arc A19 (-5.5, 47.9) -> (-5, 48.4) centre (-5.5, 48.4) ccw
  arc A20 (-13, 48.4) -> (-12.5, 47.9) centre (-12.5, 48.4) ccw
  arc A21 (-53, 48.4) -> (-52.5, 47.9) centre (-52.5, 48.4) ccw
  line L41 (-53, 48.4) -> (-53, 49.2)
  line L42 (-45, 49.2) -> (-45, 51.7)
  line L43 (-45.5, 52.2) -> (-52.5, 52.2)
  line L44 (-45.5, 47.9) -> (-52.5, 47.9)
  arc A22 (-52.5, 52.2) -> (-53, 51.7) centre (-52.5, 51.7) ccw
  line L45 (-53, 51.7) -> (-53, 49.2)
  line L46 (-45, 49.2) -> (-45, 48.4)
  arc A23 (-45, 51.7) -> (-45.5, 52.2) centre (-45.5, 51.7) ccw
  arc A24 (-45.5, 47.9) -> (-45, 48.4) centre (-45.5, 48.4) ccw
  line L47 (-53, 49.2) -> (-45, 49.2)
  line L48 (-53, 49.2) -> (-45, 49.2)
  point P0 (-5, 52.2)
  point P1 (-53, 52.2)
  dimension "d114" = 0.3
  dimension "d115" = 0.3
  dimension "d117" = 8
  dimension "d118" = 3.2
  dimension "d119" = 0.3
  dimension "d120" = 2
  dimension "d121" = 0.5
  dimension "d122" = 0.5
  dimension "d187" = 0.86
  dimension "d188" = 0.86
  dimension "d189" = 0.86
  dimension "d190" = 1.7
  dimension "d191" = 1.7
  dimension "d192" = 0.15
  dimension "d207" = 8
  dimension "d208" = 3
  dimension "d209" = 1
  dimension "d210" = 0.3
  dimension "d211" = 5
  dimension "d212" = 0.5
  dimension "d213" = 0.5
  dimension "d214" = 0.5
  dimension "d215" = 0.5
  constraint coincident L17 L20.start
  constraint coincident L19 L20.end
  constraint perpendicular L19 L20
  constraint coincident L14 L21.start
  constraint coincident L16 L21.end
  constraint perpendicular L16 L21
  constraint concentric A0 A9
  constraint concentric A9 A11
  constraint coincident A0.centre A9.centre
  constraint midpoint L4 L22.end
  constraint coincident A9 L23.end
  constraint horizontal L23
  constraint tangent A9 L24
  constraint symmetric L22 L23.end L25.start
  constraint coincident L25 L27.start
  constraint coincident L24 L27.end
  constraint perpendicular L24 L27
  constraint tangent L26 A12
  constraint tangent L25 A12
  constraint tangent L24 A13
  constraint tangent L26 A13
  constraint symmetric L22 L24 L25
  constraint coincident L9 L28.start
  constraint perpendicular L9 L28
  constraint parallel L13 L29
  constraint coincident L9 L30.start
  constraint perpendicular L9 L30
  constraint tangent L30 A14
  constraint tangent L29 A14
  constraint tangent L28 A15
  constraint tangent L29 A15
  constraint concentric A0 A16
  constraint horizontal L31
  constraint vertical L32
  constraint horizontal L33
  constraint vertical L34
  constraint horizontal L35
  constraint vertical L36
  constraint horizontal L37
  constraint vertical L38
  constraint collinear L32 L36
  constraint coincident P0 L33
  constraint coincident P0 L34
  constraint tangent L33 A17
  constraint tangent L34 A17
  constraint tangent L32 A18
  constraint tangent L33 A18
  constraint tangent L37 A19
  constraint tangent L38 A19
  constraint tangent L36 A20
  constraint tangent L37 A20
  constraint symmetric L22 L31.start L41.end
  constraint symmetric L22 L31.end L42.start
  constraint symmetric L22 P0 P1
  constraint symmetric L22 L33.end L43.end
  constraint symmetric L22 L34.start A22.end
  constraint symmetric L22 A17 A22
  constraint symmetric L22 L32.end L42.end
  constraint symmetric L22 L33.start L43.start
  constraint symmetric L22 A18 A23
  constraint symmetric L22 L37.end A21.end
  constraint symmetric L22 L38.start A21.start
  constraint symmetric L22 A19 A21
  constraint symmetric L22 L36.end L46.end
  constraint symmetric L22 L37.start L44.start
  constraint symmetric L22 A20 A24
  measures "d114" distance of L3 L20
  measures "d115" distance of L1 L21
  measures "d117" diameter of A9
  measures "d118" diameter of A11
  measures "d119" distance of L4 L27
  measures "d120" distance of L26 L27
  measures "d121" radius of A12
  measures "d122" radius of A13
  measures "d187" distance of L8 L30
  measures "d188" distance of L13 L29
  measures "d189" distance of L10 L28
  measures "d190" radius of A14
  measures "d191" radius of A15
  measures "d192" distance of A10 A16
  measures "d207" distance of L31.start L31.end
  measures "d208" distance of L31.start P0
  measures "d209" distance of L37 L39
  measures "d210" distance of L31 L39
  measures "d211" distance of L34 L40
  measures "d212" radius of A17
  measures "d213" radius of A18
  measures "d214" radius of A19
  measures "d215" radius of A20
extrude "Extrude1'" add sketch "Sketch1" along normal blind 2 separate body contours L29 L30 L32 A15 A16 L41 L46 L48 A23 L51 L52 A24 L53 | L29 L30 L32 A8 L38 A15 A16 L43 L44 L45 A19 A20 L47 L49 L50 A21 A22 L58 L59 A26 | L29 A8 L58 L59 A26 | L32 L43 L45 L46 L57 | A8 | L43 L44 L45 A19 A20 L57 | L32 L37 L38 L54 | L30 L47 L48 L49 L56 | L30 L31 L32 L37 L41 | L37 L38 L54 L55 | L47 L49 L50 A21 A22 L56 | L30 L37 L38 L55 | L39 L40 L41 L42 A17 A18 A23 L51 L52 A24 L53 | A9 | L33 L34 L35 L36 A11 A12 A13 A14 | A25 | L60 L61 L62 L63 L64 L65 A27 A28 A29 A30 A31 A32 makes body 2 in component "Versa64case_v2_top_closed"
extrude "Extrude3" add sketch "Sketch1" against normal blind 8.8 contours L29 A8 L58 L59 A26 | A8 | A25 bodies 2 in component "Versa64case_v2_top_closed"
extrude "Extrude4'" add sketch "Sketch1" against normal blind 8.8 contours L43 L44 L45 A19 A20 L57 | L37 L38 L54 L55 | L47 L49 L50 A21 A22 L56 bodies 2 in component "Versa64case_v2_top_closed"
extrude "Extrude6'" add sketch "Sketch1" against normal blind 10.4 contours L29 L30 L32 A15 A16 L41 L46 L48 A23 L51 L52 A24 L53 | L32 L43 L45 L46 L57 | L32 L37 L38 L54 | L30 L47 L48 L49 L56 | L30 L37 L38 L55 bodies 2 in component "Versa64case_v2_top_closed"
extrude "Extrude7'" add sketch "Sketch1" against normal blind 8.4 contours L39 L40 L41 L42 A17 A18 A23 L51 L52 A24 L53 bodies 2 in component "Versa64case_v2_top_closed"
extrude "Extrude8'" cut sketch "Sketch1" along normal blind 1 contours L33 L34 L35 L36 A11 A12 A13 A14 | L60 L61 L62 L63 L64 L65 A27 A28 A29 A30 A31 A32 bodies 2 in component "Versa64case_v2_top_closed"
fillet "Fillet1" radius 2 5 edges at (63, 28.7, 10.8) (62.2678, 59.1678, 10.8) (29, 59.9, 10.8) (-4.2678, 59.1678, 10.8) (-5, 28.7, 10.8) on bodies 2 in component "Versa64case_v2_top_closed"
extrude "Extrude1''" add sketch "Sketch1 (2)" along normal blind 2 separate body contours L5 L7 L9 L11 | L7 L9 L11 A2 L12 A4 L28 L29 L30 A14 A15 | L5 L6 L7 L11 | L6 L7 L11 A2 L12 A4 L14 A5 L15 A6 L16 L17 A7 L18 A8 L19 | L8 L9 L10 A1 L13 A3 L28 L29 L30 A14 A15 | L7 L14 L16 L21 | L11 L17 L19 L20 | L14 A5 L15 A6 L16 L21 | L17 A7 L18 A8 L19 L20 | A9 | A9 L24 L25 L39 | L24 L25 L27 L39 | L24 L25 L26 L27 A12 A13 | A16 | L31 L35 L36 L38 L39 | L31 L32 L33 L34 L35 A17 A18 | L36 L37 L38 L39 A19 A20 | L39 A21 L41 L44 L46 A24 | L39 L41 L46 L47 L48 | L42 L43 A22 L45 A23 L47 L48 makes body 3 in component "versa64case_v2_bottom_closed"
extrude "Extrude2'" add sketch "Sketch1 (2)" against normal blind 6.5 contours L5 L6 L7 L11 | L14 A5 L15 A6 L16 L21 | L17 A7 L18 A8 L19 L20 | A9 | A9 L24 L25 L39 | L24 L25 L27 L39 | L31 L35 L36 L38 L39 | L36 L37 L38 L39 A19 A20 | L39 A21 L41 L44 L46 A24 | L39 L41 L46 L47 L48 bodies 3 in component "versa64case_v2_bottom_closed"
extrude "Extrude6''" add sketch "Sketch1 (2)" against normal blind 8.1 contours A16 bodies 3 in component "versa64case_v2_bottom_closed"
chamfer "Chamfer2" distance 0.3 angle 45 1 edges at (31.191, 44.7498, 0) on bodies 3 in component "versa64case_v2_bottom_closed"
extrude "Extrude7''" add sketch "Sketch1 (2)" against normal blind 6.5 contours L7 L9 L11 A2 L12 A4 L28 L29 L30 A14 A15 | L7 L14 L16 L21 | L11 L17 L19 L20 bodies 3 in component "versa64case_v2_bottom_closed"
extrude "Extrude4''" add sketch "Sketch1 (2)" against normal blind 8.5 contours L8 L9 L10 A1 L13 A3 L28 L29 L30 A14 A15 bodies 3 in component "versa64case_v2_bottom_closed"
extrude "Extrude5'" add sketch "Sketch1 (2)" against normal blind 8.1 contours L24 L25 L26 L27 A12 A13 | L31 L32 L33 L34 L35 A17 A18 | L42 L43 A22 L45 A23 L47 L48 bodies 3 in component "versa64case_v2_bottom_closed"
fillet "Fillet4" radius 0.5 8 edges at (61, 37.9, 3.6) (61, 35.9, 3.6) (61, 11.5, 3.6) (61, 9.5, 3.6) (-3, 33.3, 3.6) (-3, 35.3, 3.6) (-3, 11.5, 3.6) (-3, 9.5, 3.6) on bodies 2 in component "Versa64case_v2_top_closed"
fillet "Fillet12" radius 0.8 1 edges at (32, 57.9, 4.4) on bodies 2 in component "Versa64case_v2_top_closed"
fillet "Fillet5" radius 0.5 30 edges at (-3, 4.5, 8.8) (-2.8536, 9.3536, 8.8) (29, 9.5, 8.8) (60.8536, 9.3536, 8.8) (61, 4.5, 8.8) (-2.8536, 11.6464, 8.8) (-3, 22.4, 8.8) (-2.8536, 33.1536, 8.8) (-0.5, 33.3, 8.8) (1.8536, 33.4464, 8.8) (2, 34.3, 8.8) (1.8536, 35.1536, 8.8) (-0.5, 35.3, 8.8) (-2.8536, 35.4464, 8.8) (-3, 46.6, 8.8) (-2.8536, 57.7536, 8.8) (46.25, 57.9, 8.8) (10.25, 57.9, 8.8) (60.8536, 57.7536, 8.8) (61, 47.9, 8.8) (60.8536, 38.0464, 8.8) (58.5, 37.9, 8.8) (56.1464, 37.7536, 8.8) (56, 36.9, 8.8) (56.1464, 36.0464, 8.8) (58.5, 35.9, 8.8) (60.8536, 35.7536, 8.8) (61, 23.7, 8.8) (60.8536, 11.6464, 8.8) (29, 11.5, 8.8) on bodies 2 in component "Versa64case_v2_top_closed"
fillet "Fillet7" radius 0.5 5 edges at (-3, 0, 3.35) (-2.8536, 0, 8.6536) (29, 0, 8.8) (60.8536, 0, 8.6536) (61, 0, 3.35) on bodies 2 in component "Versa64case_v2_top_closed"
fillet "Fillet8" radius 0.5 5 edges at (63, 0, 4.6) (62.4142, 0, 10.2142) (29, 0, 10.8) (-4.4142, 0, 10.2142) (-5, 0, 4.6) on bodies 2 in component "Versa64case_v2_top_closed"